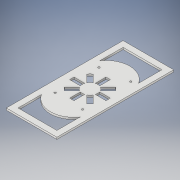
# Autodesk Inventor part: Cuerpo - Base
Saved by Autodesk Inventor 2019 (Build 230136000, 136)
## iProperties
Created: 2020-02-15
Part Number: Cuerpo - Base
Material: ABS Plastic
Document SubType Name: Modeling
Designer: Mafer1
Density: 1.06 g/cm^3
Appearance: Smooth - White
Mass: 43.8755 g
Surface Area: 296.565 cm^2
Volume: 41.392 cm^3
ancho_base: 80.000 mm
largo_base: 200.000 mm
Author: Mafer1
Autodesk Inventor part; units mm, degrees
ref_plane "YZ Plane" through (0, 0, 0) normal (1, 0, 0) x (0, 1, 0)
ref_plane "XZ Plane" through (0, 0, 0) normal (0, 1, 0) x (-1, 0, 0)
ref_plane "XY Plane" through (0, 0, 0) normal (0, 0, 1) x (1, 0, 0)
sketch "Boceto1" plane through (0, 0, 0) normal (0, 1, 0) x (-1, 0, 0)
  line L0 (0, 0) -> (86.6, 0)
  line L1 (86.6, 0) -> (86.6, -200)
  line L2 (86.6, -200) -> (0, -200)
  line L3 (0, -200) -> (0, 0)
  dimension "d0" = 200
  dimension "d1" = 86.6
  constraints: 8 end point, 2 parallel, 1 horizontal, 1 perpendicular
  measures "d0" distance of L0.end L1.end
  measures "d1" distance between parallel lines of L3 L1
extrude "Extrusión1" add sketch "Boceto1" along normal blind 3.3
sketch "Boceto2" plane through (0, 3.3, 0) normal (0, 1, 0) x (1, 0, 0)
  circle A0 centre (-43.3, 100) radius 13.3 construction
  circle A1 centre (-43.3, 100) radius 31.3 construction
  line L0 (-86.6, 0) -> (0, 0) projected
  line L1 (0, 0) -> (0, 200) projected
  line L2 (0, 200) -> (-86.6, 200) projected
  line L3 (-86.6, 200) -> (-86.6, 0) projected
  line L4 (0, 200) -> (-86.6, 200) projected
  line L5 (-47.05, 68.9255) -> (-47.05, 87.2396)
  line L6 (-39.55, 68.9255) -> (-39.55, 87.2396)
  arc A2 (-47.05, 87.2396) -> (-39.55, 87.2396) centre (-43.3, 100) ccw
  arc A3 (-47.05, 68.9255) -> (-39.55, 68.9255) centre (-43.3, 100) ccw
  line L7 (-18.6753, 80.6786) -> (-31.6254, 93.6287)
  arc A4 (-23.9786, 75.3753) -> (-18.6753, 80.6786) centre (-43.3, 100) ccw
  line L8 (-23.9786, 75.3753) -> (-36.9287, 88.3254)
  arc A5 (-36.9287, 88.3254) -> (-31.6254, 93.6287) centre (-43.3, 100) ccw
  line L9 (-12.2255, 103.75) -> (-30.5396, 103.75)
  arc A6 (-12.2255, 96.25) -> (-12.2255, 103.75) centre (-43.3, 100) ccw
  line L10 (-12.2255, 96.25) -> (-30.5396, 96.25)
  arc A7 (-30.5396, 96.25) -> (-30.5396, 103.75) centre (-43.3, 100) ccw
  line L11 (-23.9786, 124.6247) -> (-36.9287, 111.6746)
  arc A8 (-18.6753, 119.3214) -> (-23.9786, 124.6247) centre (-43.3, 100) ccw
  line L12 (-18.6753, 119.3214) -> (-31.6254, 106.3713)
  arc A9 (-31.6254, 106.3713) -> (-36.9287, 111.6746) centre (-43.3, 100) ccw
  line L13 (-47.05, 131.0745) -> (-47.05, 112.7604)
  arc A10 (-39.55, 131.0745) -> (-47.05, 131.0745) centre (-43.3, 100) ccw
  line L14 (-39.55, 131.0745) -> (-39.55, 112.7604)
  arc A11 (-39.55, 112.7604) -> (-47.05, 112.7604) centre (-43.3, 100) ccw
  line L15 (-67.9247, 119.3214) -> (-54.9746, 106.3713)
  arc A12 (-62.6214, 124.6247) -> (-67.9247, 119.3214) centre (-43.3, 100) ccw
  line L16 (-62.6214, 124.6247) -> (-49.6713, 111.6746)
  arc A13 (-49.6713, 111.6746) -> (-54.9746, 106.3713) centre (-43.3, 100) ccw
  line L17 (-74.3745, 96.25) -> (-56.0604, 96.25)
  arc A14 (-74.3745, 103.75) -> (-74.3745, 96.25) centre (-43.3, 100) ccw
  line L18 (-74.3745, 103.75) -> (-56.0604, 103.75)
  arc A15 (-56.0604, 103.75) -> (-56.0604, 96.25) centre (-43.3, 100) ccw
  line L19 (-62.6214, 75.3753) -> (-49.6713, 88.3254)
  arc A16 (-67.9247, 80.6786) -> (-62.6214, 75.3753) centre (-43.3, 100) ccw
  line L20 (-67.9247, 80.6786) -> (-54.9746, 93.6287)
  arc A17 (-54.9746, 93.6287) -> (-49.6713, 88.3254) centre (-43.3, 100) ccw
  line L21 (-86.6, 200) -> (-86.6, 0) projected
  line L22 (0, 0) -> (0, 200) projected
  point P0 (-43.3, 200)
  point P1 (-86.6, 100)
  point P2 (-43.3, 200)
  point P3 (-43.3, 86.7)
  point P4 (-33.8955, 90.5955)
  point P5 (-30, 100)
  point P6 (-33.8955, 109.4045)
  point P7 (-43.3, 113.3)
  point P8 (-52.7045, 109.4045)
  point P9 (-56.6, 100)
  point P10 (-52.7045, 90.5955)
  dimension "d10" = 18
  dimension "d11" = 7.5
  dimension "d14" = 360
  dimension "d19" = 30
  constraints: 37 point on circle, 32 end point, 18 centre point, 3 midpoint, 3 parallel, 3 vertical alignment, 2 concentric, 1 coincident, 1 horizontal alignment, 1 vertical, 89 other
  measures "d10" radial gap between concentric circles of A1 A0
  measures "d11" distance between parallel lines of L6 L5
  measures "d19" distance of point (-86.6, 100) point (-56.6, 100)
extrude "Extrusión2" cut sketch "Boceto2" against normal blind 10 contours L5 A2 L6 A3 | A4 L8 A5 L7 | A6 L10 A7 L9 | A8 L12 A9 L11 | A10 L14 A11 L13 | A12 L16 A13 L15 | A14 L18 A15 L17 | A16 L20 A17 L19
sketch "Sketch3" plane through (0, 3.3, 0) normal (0, 1, 0) x (1, 0, 0)
  line L0 (-86.6, 200) -> (-86.6, 0) projected
  line L1 (-69.975, 150.795) -> (-16.625, 150.795) construction
  line L2 (-16.625, 150.795) -> (-16.625, 49.205) construction
  line L3 (-16.625, 49.205) -> (-69.975, 49.205) construction
  line L4 (-69.975, 49.205) -> (-69.975, 150.795) construction
  line L5 (0, 200) -> (-86.6, 200) projected
  circle A0 centre (-67.425, 64.445) radius 1.5875
  circle A1 centre (-19.165, 63.175) radius 1.5875
  circle A2 centre (-19.165, 145.725) radius 1.5875
  circle A3 centre (-67.425, 139.375) radius 1.5875
  circle A4 centre (-24.245, 115.245) radius 1.5875
  point P0 (0, 0)
  dimension "d21" = 101.59
  dimension "d22" = 53.35
  dimension "d23" = 16.625
  dimension "d24" = 49.205
  dimension "d25" = 15.24
  dimension "d26" = 3.175
  dimension "d28" = 50.8
  dimension "d29" = 13.97
  dimension "d30" = 2.54
  dimension "d31" = 90.17
  dimension "d32" = 96.52
  dimension "d34" = 50.8
  dimension "d35" = 2.54
  dimension "d36" = 66.04
  dimension "d37" = 7.62
  constraints: 8 end point, 5 centre point, 4 equal radius, 2 parallel, 1 horizontal, 1 perpendicular
  measures "d21" distance of L1.end L2.end
  measures "d22" distance of L2.end L3.end
  measures "d23" distance between parallel lines of L4 L0
  measures "d24" distance between parallel lines of L1 L5
  measures "d25" distance from line of L3 A0.centre
  measures "d26" diameter of A0
  measures "d28" distance from line of A0.centre L2
  measures "d29" distance from line of L3 A1.centre
  measures "d30" distance from line of A1.centre L2
  measures "d31" distance from line of A3.centre L3
  measures "d32" distance from line of A2.centre L3
  measures "d34" distance from line of A3.centre L2
  measures "d35" distance from line of A2.centre L2
  measures "d36" distance from line of A4.centre L3
  measures "d37" distance from line of A4.centre L2
extrude "Extrusion3" cut sketch "Sketch3" against normal blind 10 contours A0 | A1 | A2 | A3
sketch "Sketch4" plane through (0, 3.3, 0) normal (0, 1, 0) x (1, 0, 0)
  line L0 (-10, 10) -> (-76.6, 10)
  line L1 (-76.6, 10) -> (-76.6, 50)
  line L2 (-10, 10) -> (-10, 50)
  arc A0 (-76.6, 50) -> (-10, 50) centre (-43.3, 72.161) ccw
  line L3 (-86.6, 0) -> (0, 0) projected
  line L4 (-86.6, 200) -> (-86.6, 0) projected
  line L5 (0, 0) -> (0, 200) projected
  dimension "d40" = 10
  dimension "d41" = 10
  dimension "d42" = 10
  dimension "d43" = 40
  dimension "d44" = 40
  constraints: 6 end point, 2 point on circle, 1 centre point, 1 horizontal, 1 parallel, 1 perpendicular, 1 vertical
  measures "d40" distance between parallel lines of L3 L0
  measures "d41" distance between parallel lines of L4 L1
  measures "d42" distance between parallel lines of L5 L2
  measures "d43" distance of L0.start L2.end
  measures "d44" radius of A0
ref_plane "Work Plane1" through (0, 0, -100) normal (0, 0, -1) x (-1, 0, 0)
extrude "Extrusion4" cut sketch "Sketch4" against normal blind 10
mirror "Mirror1" about plane through (0, 0, -100) normal (0, 0, -1) of "Extrusion4"
equation "\"d0\" = largo_base"
equation "\"d10\" = 1.5 * d4"
equation "\"d11\" = 0.25 * d19"
equation "\"d19\" = d8"
equation "\"d24\" = 0.5 * largo_base - 0.5 * d21"
equation "\"d34\" = d28"
equation "\"d35\" = d30"
equation "\"ancho_base\" = 80"
equation "\"largo_base\" = 200"
equation "\"d4\" = 12"
equation "\"d8\" = 30"
